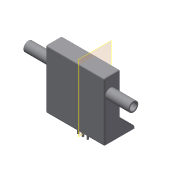
# Autodesk Inventor part: AWM3100
Saved by Autodesk Inventor 2019 (Build 230136000, 136)
## iProperties
Created: 2021-03-03
Part Number: AWM3100
Material: Generic
Document SubType Name: Modeling
Designer: LuoYi
Density: 1 g/cm^3
Appearance: Smooth - Light Orange
Author: LuoYi
Autodesk Inventor part; units mm, degrees
ref_plane "YZ Plane" through (0, 0, 0) normal (1, 0, 0) x (0, 1, 0)
ref_plane "XZ Plane" through (0, 0, 0) normal (0, 1, 0) x (-1, 0, 0)
ref_plane "XY Plane" through (0, 0, 0) normal (0, 0, 1) x (1, 0, 0)
sketch "Sketch1" plane through (0, 0, 0) normal (0, 0, 1) x (1, 0, 0)
  line L0 (0, 0) -> (30.5, 0)
  line L1 (30.5, 0) -> (30.5, 30.5)
  line L2 (30.5, 30.5) -> (0, 30.5)
  line L3 (0, 30.5) -> (0, 0)
  dimension "d0" = 30.5
  dimension "d1" = 30.5
  constraints: 8 end point, 2 parallel, 1 horizontal, 1 perpendicular
  measures "d0" distance of L2.end L1.end
  measures "d1" distance of L1.end L0.end
extrude "Extrusion1" add sketch "Sketch1" along normal blind 8.25
sketch "Sketch3" plane through (0, 0, 0) normal (0, -1, 0) x (1, 0, 0)
  line L0 (30.5, 0) -> (30.5, 8.25) projected
  line L1 (30.5, 5.45) -> (0, 5.45)
  line L2 (0, 5.45) -> (0, -7.25)
  line L3 (0, -7.25) -> (30.5, -7.25)
  line L4 (30.5, -7.25) -> (30.5, 5.45)
  line L5 (0, 8.25) -> (30.5, 8.25) projected
  point P0 (0, 0)
  dimension "d6" = 15.5
  dimension "d7" = 12.7
  constraints: 8 end point, 2 parallel, 1 horizontal, 1 perpendicular, 1 point on line
  measures "d6" distance between parallel lines of L3 L5
  measures "d7" distance between parallel lines of L1 L3
extrude "Extrusion2" add sketch "Sketch3" against normal blind 1.8
sketch "Sketch4" plane through (30.5, 0, 0) normal (1, 0, 0) x (0, 0, -1)
  line L0 (0, 1.8) -> (0, 30.5) projected
  line L1 (0, 1.8) -> (7.25, 1.8)
  line L2 (7.25, 1.8) -> (0, 9.05)
  line L3 (0, 1.8) -> (7.25, 1.8) projected
  line L4 (7.25, 1.8) -> (0, 1.8) projected
  line L5 (0, 9.05) -> (0, 1.8)
  line L6 (7.25, 0) -> (7.25, 1.8) projected
  point P0 (0, 0)
  dimension "d10" = 45
  constraints: 6 end point, 2 point on line, 1 collinear, 1 horizontal, 1 perpendicular
  measures "d10" angle of L1 L2
extrude "Extrusion3" add sketch "Sketch4" against normal blind 1.8
ref_plane "Work Plane1" through (17.65, 0, 8.25) normal (1, 0, 0) x (0, 0, -1)
sketch "Sketch5" plane through (17.65, 0, 8.25) normal (1, 0, 0) x (0, 0, -1)
  line L0 (15.5, 1.8) -> (8.25, 9.05) projected
  line L1 (8.25, 9.05) -> (8.25, 1.8) projected
  line L2 (8.25, 1.8) -> (15.5, 1.8) projected
  point P0 (8.25, 0)
extrude "Extrusion4" add sketch "Sketch5" against normal blind 1.8
sketch "Sketch6" plane through (0, 0, 8.25) normal (-1, 0, 0) x (0, 0, 1)
  line L0 (-8.25, 9.05) -> (-15.5, 1.8) projected
  line L1 (-8.25, 1.8) -> (-15.5, 1.8) projected
  line L2 (-8.25, 9.05) -> (-8.25, 1.8) projected
  point P0 (-8.25, 0)
extrude "Extrusion5" add sketch "Sketch6" against normal blind 1.8
sketch "Sketch9" plane through (0, 1.8, 0) normal (0, 1, 0) x (1, 0, 0)
  circle A0 centre (23.15, 3.15) radius 1.45
  line L0 (7.65, 3.15) -> (10.45, 3.15) construction
  line L1 (7.65, 1.75) -> (10.45, 1.75)
  line L2 (10.45, 4.55) -> (7.65, 4.55)
  arc A1 (7.65, 4.55) -> (7.65, 1.75) centre (7.65, 3.15) ccw
  arc A2 (10.45, 1.75) -> (10.45, 4.55) centre (10.45, 3.15) ccw
  line L3 (17.65, 7.25) -> (15.85, 7.25) projected
  line L4 (16.75, 7.25) -> (16.75, -1.0968) construction
  line L5 (15.85, 0) -> (15.85, 7.25) projected
  line L6 (28.7, 7.25) -> (17.65, 7.25) projected
  point P0 (0, 0)
  point P1 (9.05, 3.15)
  dimension "d30" = 2.9
  dimension "d31" = 1.4
  dimension "d32" = 2.8
  dimension "d33" = 12.7
  dimension "d34" = 6.4
  dimension "d35" = 4.1
  constraints: 10 end point, 4 point on circle, 4 tangent, 3 centre point, 2 midpoint, 2 parallel, 1 horizontal, 1 point on line
  measures "d30" diameter of A0
  measures "d31" radius of A2
  measures "d32" distance of L2.start L2.end
  measures "d33" distance of A0.centre L0.end
  measures "d34" distance from line of A0.centre L4
  measures "d35" distance from line of L6 A0.centre
extrude "Extrusion6" cut sketch "Sketch9" against normal blind 1.8
sketch "Sketch8" plane through (0, 0, 8.25) normal (0, -1, 0) x (1, 0, 0)
  line L0 (13.065, -4.425) -> (12.435, -4.425)
  line L1 (12.435, -4.425) -> (12.435, -3.795)
  line L2 (12.435, -3.795) -> (13.065, -3.795)
  line L3 (13.065, -3.795) -> (13.065, -4.425)
  line L4 (13.065, -4.425) -> (12.435, -3.795) construction
  line L5 (12.435, -4.425) -> (13.065, -3.795) construction
  line L6 (15.565, -4.425) -> (14.935, -4.425)
  line L7 (14.935, -4.425) -> (14.935, -3.795)
  line L8 (14.935, -3.795) -> (15.565, -3.795)
  line L9 (15.565, -3.795) -> (15.565, -4.425)
  line L10 (15.565, -4.425) -> (14.935, -3.795) construction
  line L11 (14.935, -4.425) -> (15.565, -3.795) construction
  line L12 (18.065, -4.425) -> (17.435, -4.425)
  line L13 (17.435, -4.425) -> (17.435, -3.795)
  line L14 (17.435, -3.795) -> (18.065, -3.795)
  line L15 (18.065, -3.795) -> (18.065, -4.425)
  line L16 (18.065, -4.425) -> (17.435, -3.795) construction
  line L17 (17.435, -4.425) -> (18.065, -3.795) construction
  line L18 (0, 0) -> (30.5, 0) projected
  line L19 (15.25, 0) -> (15.25, -15.5) construction
  line L20 (15.85, -15.5) -> (1.8, -15.5) projected
  circle A0 centre (23.15, -11.4) radius 1.45 projected
  point P0 (0, -8.25)
  point P1 (12.75, -4.11)
  point P2 (15.25, -4.11)
  point P3 (17.75, -4.11)
  point P4 (15.25, -4.11)
  dimension "d23" = 0.63
  dimension "d24" = 0.63
  dimension "d25" = 0.63
  dimension "d26" = 0.63
  dimension "d27" = 0.63
  dimension "d28" = 2.5
  dimension "d29" = 2.5
  dimension "d38" = 7.29
  constraints: 38 end point, 8 midpoint, 6 parallel, 3 collinear, 3 horizontal, 3 perpendicular, 2 point on line, 1 vertical
  measures "d23" distance of L1.end L2.end
  measures "d24" distance of L2.end L0.start
  measures "d25" distance of L7.end L8.end
  measures "d26" distance of L13.end L14.end
  measures "d27" distance of L12.end L13.end
  measures "d28" distance of point (15.25, -4.11) point (12.75, -4.11)
  measures "d29" distance of point (17.75, -4.11) point (15.25, -4.11)
  measures "d38" vertical distance of point (17.75, -4.11) A0.centre
extrude "Extrusion7" add sketch "Sketch8" along normal blind 5.1 contours L0 L1 L2 L3 | L6 L7 L8 L9 | L12 L13 L14 L15
sketch "Sketch7" plane through (0, 0, 8.25) normal (0, -1, 0) x (1, 0, 0)
  line L0 (15.85, -15.5) -> (1.8, -15.5) projected
  line L1 (2.55, -15.5) -> (4.05, -15.5)
  line L2 (4.05, -15.5) -> (4.05, -2.8)
  line L3 (4.05, -2.8) -> (2.55, -2.8)
  line L4 (2.55, -2.8) -> (2.55, -15.5)
  line L5 (28.7, -15.5) -> (17.65, -15.5) projected
  line L6 (27.95, -15.5) -> (26.45, -15.5)
  line L7 (26.45, -15.5) -> (26.45, -2.8)
  line L8 (26.45, -2.8) -> (27.95, -2.8)
  line L9 (27.95, -2.8) -> (27.95, -15.5)
  line L10 (13.25, -2.8) -> (14.75, -2.8)
  line L11 (14.75, -2.8) -> (14.75, -15.5)
  line L12 (14.75, -15.5) -> (13.25, -15.5)
  line L13 (13.25, -15.5) -> (13.25, -2.8)
  line L14 (3.3, -2.8) -> (3.3, -15.5) construction
  line L15 (27.2, -2.8) -> (27.2, -15.5) construction
  line L16 (0, 0) -> (30.5, 0) projected
  line L17 (15.25, 0) -> (15.25, -15.5) construction
  line L18 (14, -2.8) -> (14, -15.5) construction
  line L19 (14.935, -3.795) -> (14.935, -4.425) projected
  line L20 (14.935, -4.11) -> (13.065, -4.11) construction
  line L21 (13.065, -3.795) -> (13.065, -4.425) projected
  point P0 (0, -8.25)
  point P1 (14, -4.11)
  dimension "d18" = 1.5
  dimension "d19" = 1.5
  dimension "d20" = 1.5
  dimension "d21" = 23.9
  dimension "d22" = 12.7
  constraints: 34 end point, 10 midpoint, 6 parallel, 6 point on line, 5 perpendicular, 3 horizontal, 1 collinear, 1 other
  measures "d18" distance between parallel lines of L4 L2
  measures "d19" distance between parallel lines of L9 L7
  measures "d20" distance between parallel lines of L11 L13
  measures "d21" distance between parallel lines of L15 L14
  measures "d22" distance between parallel lines of L0 L3
extrude "Extrusion8" add sketch "Sketch7" along normal blind 1
sketch "Sketch2" plane through (30.5, 0, 0) normal (1, 0, 0) x (0, 0, -1)
  circle A0 centre (-5.25, 22.4) radius 2.55
  circle A1 centre (-5.25, 22.4) radius 1.8
  line L0 (7.25, -1) -> (-5.45, -1) projected
  line L1 (1.7, 1.8) -> (4.6, 1.8) projected
  point P0 (0, 0)
  point P1 (3.15, 1.8)
  dimension "d4" = 5.1
  dimension "d5" = 3.6
  dimension "d44" = 23.4
  dimension "d45" = 8.4
  constraints: 2 centre point, 1 coincident, 1 midpoint
  measures "d4" diameter of A0
  measures "d5" diameter of A1
  measures "d44" distance from line of L0 A0.centre
  measures "d45" horizontal distance of A0.centre point (3.15, 1.8)
extrude "Extrusion9" add sketch "Sketch2" along normal blind 11.95
sketch "Sketch10" plane through (0, 0, 8.25) normal (-1, 0, 0) x (0, 0, 1)
  circle A0 centre (-3, 22.4) radius 1.8 projected
  circle A1 centre (-3, 22.4) radius 2.55 projected
  point P0 (-8.25, 0)
extrude "Extrusion10" add sketch "Sketch10" along normal blind 11.95
fillet "Fillet1" radius 0.7 17 edges at (30.5, 30.5, 4.125) (15.25, 30.5, 8.25) (30.5, 15.25, 8.25) (30.5, 0, 0.5) (15.25, 0, 8.25) (0, 15.25, 8.25) (0, 30.5, 4.125) (15.25, 30.5, 0) (0, 0, 0.5) (30.5, 19.775, 0) (0, 19.775, 0) (30.5, 5.425, -3.625) (28.7, 5.425, -3.625) (17.65, 5.425, -3.625) (15.85, 5.425, -3.625) (1.8, 5.425, -3.625) (0, 5.425, -3.625)
body "Solid1"
